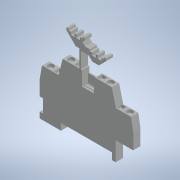
# Autodesk Inventor part: 280-519_LO
Saved by Autodesk Inventor 2021 (Build 250183000, 183)
## iProperties
Created: 2026-07-31
Part Number: 280-519_LO
Material: Generic
Catalog Web Link: www.3dfindit.com
Description: 280-519-Double-deck terminal block, Through/through terminal block, for DIN-rail 35 x 15 and 35 x 7.5, 2.5 mm², CAGE CLAMP®
Vendor: WAGO
Document SubType Name: Modeling
Designer: psAdmin
Manufacturer: WAGO
Mass: 10.061 g
Surface Area: 63.9443 cm^2
Volume: 10.5778 cm^3
Density: 1 g/cm^3
Appearance: PSOLRGB-143-145-145
Category: PARTsolutions
Company: WAGO
Title: 280-519
Author: Cadenas PARTsolutions
Comments: Double-deck terminal block, Through/through terminal block, for DIN-rail 35 x 15 and 35 x 7.5, 2.5 mm², CAGE CLAMP®
PSOL_IDENT_0: {$CADENAS_DATA/23d-libs/wago/pg01/serie280/0280-0519_0999-0962.prj},163 {VTYP=3D},{NB=280-519_LO},{L
PSOL_IDENT_1: INA=280-519},{NN=280-519},{DATE=07.07.2026 10:57:29},{GEOMDATE=12.11.2024 14:37:53},{VERSION=},{LINE
PSOL_IDENT_2: ID=2570},{WBVAR=LOD},{WBNUMERIC=}  {NB=280-519_LO},{LINA=280-519},{KT=DUMMY},{BESTNR=280-519},{INFOD
PSOL_IDENT_3: E=Info DE},{INFOEN=Info EN},{LOD=LO},{QUERSCHNITT1=0.08 - 2.5},{QUERSCHNITT2=28 - 12},{ABISOLIERLAEN
PSOL_IDENT_4: GE=8 - 9},{SPANNUNG=500},{BEMESSSTOSSSPG=6},{VERSCHMUTZGRAD=3},{STROM=20},{HOEHE=58.50},{BREITE=5.00
PSOL_IDENT_5: },{TIEFE=64.00},{ANZAHLKLEMMSTEL=4},{ANZAHLPOTENTIAL=2},{FARBE=grau},{BEMERKUNGEN=},{RGB=0.56,0.57,0
PSOL_IDENT_6: .57,0},{GEWICHT=10.061},{ECLASS71=27-14-11-20},{LINKDE=http://www.wago.com/de/p/280-519},{LINKEN=htt
PSOL_IDENT_7: p://www.wago.com/global/p/280-519},{FILENAME=280-519}
NB: 280-519_LO
NN: 280-519
NT: Double-deck terminal block, Through/through terminal block, for DIN-rail 35 x 15 and 35 x 7.5, 2.5 mm², CAGE CLAMP®
NBSYN: $BESTNR._$LOD.
LINA: 280-519
CATALOG: WAGO
OFFICIAL_STANDARD_NUMBERS: NO
BESTNR: 280-519
INFODE: Info DE
INFOEN: Info EN
LOD: LOW
QUERSCHNITT1: 0.08 - 2.5
QUERSCHNITT2: 28 - 12
ABISOLIERLAENGE: 8 - 9
SPANNUNG: 500
BEMESSSTOSSSPG: 6
VERSCHMUTZGRAD: 3
STROM: 20
HOEHE: 58.5
BREITE: 5
TIEFE: 64
ANZAHLKLEMMSTEL: 4
ANZAHLPOTENTIAL: 2
FARBE: gray
GEWICHT: 10.061
ECLASS71: 27-14-11-20
SUPPLIER: WAGO
ARTICLENO: 280-519_LO
BOMINFO: 280-519
CREATOR: CADENAS GmbH
Autodesk Inventor part; units mm, degrees
sketch "Sketch_1" plane through (0, 0, 0) normal (0, 0, 1) x (1, 0, 0)
  line L0 (-32.2, -0.6) -> (-32.2, -4.6)
  line L1 (-32.2, -4.6) -> (-17.5, -4.6)
  line L2 (-17.5, -4.6) -> (-17.5, 0)
  line L3 (-17.5, 0) -> (17.5, 0)
  line L4 (17.5, 0) -> (17.5, -4.6)
  line L5 (17.5, -4.6) -> (20, -4.6)
  line L6 (20, -4.6) -> (20, 8.5)
  line L7 (20, 8.5) -> (32, 8.5)
  line L8 (32, 8.5) -> (32, 19.1)
  line L9 (32, 19.1) -> (30.5012, 27.6)
  line L10 (30.5012, 27.6) -> (-30.5012, 27.6)
  line L11 (-30.5012, 27.6) -> (-32, 19.1)
  line L12 (-32, 19.1) -> (-32, 8.5)
  line L13 (-32, 8.5) -> (-29.7, 8.5)
  line L14 (-29.7, 8.5) -> (-29.7, -0.6)
  line L15 (-29.7, -0.6) -> (-32.2, -0.6)
  constraints: 32 end point
extrude "Extrusion1" add sketch "Sketch_1" along normal blind 5
sketch "Sketch_2" plane through (0, 0, 0) normal (0, 0, 1) x (1, 0, 0)
  line L0 (-19.1, 27.6) -> (-18.2, 27.6)
  line L1 (-18.2, 27.6) -> (-18.2, 15.1)
  line L2 (-18.2, 15.1) -> (19.2, 15.1)
  line L3 (19.2, 15.1) -> (19.2, 27.6)
  line L4 (19.2, 27.6) -> (20.1, 27.6)
  line L5 (20.1, 27.6) -> (17.3574, 38.6)
  line L6 (17.3574, 38.6) -> (5.7574, 38.6)
  line L7 (5.7574, 38.6) -> (4.9, 28.8)
  line L8 (4.9, 28.8) -> (-3.1, 28.8)
  line L9 (-3.1, 28.8) -> (-3.1, 38.6)
  line L10 (-3.1, 38.6) -> (-16.3574, 38.6)
  line L11 (-16.3574, 38.6) -> (-19.1, 27.6)
  constraints: 24 end point
extrude "Extrusion2" add sketch "Sketch_2" along normal blind 5
sketch "Skizze_3" plane through (0, 0, 0) normal (0, 0, 1) x (1, 0, 0)
  line L0 (-3.1, 34.8) -> (-3.1, 28.8)
  line L1 (-3.1, 28.8) -> (5.9, 28.8)
  line L2 (5.9, 28.8) -> (5.9, 34.8)
  line L3 (5.9, 34.8) -> (-3.1, 34.8)
  constraints: 8 end point
extrude "Extrusion3" add sketch "Skizze_3" along normal blind 0.8
sketch "Sketch_3" plane through (0.5, 0, 0) normal (1, 0, 0) x (0, 0, -1)
  line L0 (-4.7, 28.4) -> (-3.3, 28.4)
  line L1 (-3.3, 28.4) -> (-3.3, 28.8)
  line L2 (-3.3, 28.8) -> (-2.5, 28.8)
  line L3 (-2.5, 28.8) -> (-2.5, 28.4)
  line L4 (-2.5, 28.4) -> (-1.1, 28.4)
  line L5 (-1.1, 28.4) -> (-1.1, 29.8)
  line L6 (-1.1, 29.8) -> (-4.7, 29.8)
  line L7 (-4.7, 29.8) -> (-4.7, 28.4)
  constraints: 16 end point
extrude "Extrusion4" cut sketch "Sketch_3" along normal mid plane 7.2
sketch "Sketch_4" plane through (0, 0, 2.5) normal (0, 0, 1) x (1, 0, 0)
  line L0 (27.1, 25.6) -> (27.1, 27.6)
  line L1 (27.1, 27.6) -> (29.2, 27.6)
  line L2 (29.2, 27.6) -> (29.2, 25.6)
  line L3 (29.2, 25.6) -> (27.1, 25.6)
  line L4 (27.1, 25.6) -> (27.1, 27.6)
  constraints: 10 end point
revolve "Revolution1" cut sketch "Sketch_4" angle 360 about axis through (27.1, 25.6, 2.5) along (0, -1, 0)
sketch "Sketch_5" plane through (0, 0, 2.5) normal (0, 0, 1) x (1, 0, 0)
  line L0 (-27.1, 25.6) -> (-27.1, 27.6)
  line L1 (-27.1, 27.6) -> (-25, 27.6)
  line L2 (-25, 27.6) -> (-25, 25.6)
  line L3 (-25, 25.6) -> (-27.1, 25.6)
  line L4 (-27.1, 25.6) -> (-27.1, 27.6)
  constraints: 10 end point
revolve "Revolution2" cut sketch "Sketch_5" angle 360 about axis through (-27.1, 25.6, 2.5) along (0, -1, 0)
sketch "Sketch_6" plane through (0, 0, 2.5) normal (0, 0, 1) x (1, 0, 0)
  line L0 (14.05, 36.6) -> (14.05, 38.6)
  line L1 (14.05, 38.6) -> (16.15, 38.6)
  line L2 (16.15, 38.6) -> (16.15, 36.6)
  line L3 (16.15, 36.6) -> (14.05, 36.6)
  line L4 (14.05, 36.6) -> (14.05, 38.6)
  constraints: 10 end point
revolve "Revolution3" cut sketch "Sketch_6" angle 360 about axis through (14.05, 36.6, 2.5) along (0, -1, 0)
sketch "Sketch_7" plane through (0, 0, 2.5) normal (0, 0, 1) x (1, 0, 0)
  line L0 (-13.05, 36.6) -> (-13.05, 38.6)
  line L1 (-13.05, 38.6) -> (-10.95, 38.6)
  line L2 (-10.95, 38.6) -> (-10.95, 36.6)
  line L3 (-10.95, 36.6) -> (-13.05, 36.6)
  line L4 (-13.05, 36.6) -> (-13.05, 38.6)
  constraints: 10 end point
revolve "Revolution4" cut sketch "Sketch_7" angle 360 about axis through (-13.05, 36.6, 2.5) along (0, -1, 0)
sketch "Skizze_15" plane through (0, 0, 2.5) normal (0, 0, 1) x (1, 0, 0)
  line L0 (-4.9, 36.6) -> (-3.9, 36.6)
  line L1 (-3.9, 36.6) -> (-3.9, 38.6)
  line L2 (-3.9, 38.6) -> (-4.9, 38.6)
  line L3 (-4.9, 38.6) -> (-4.9, 36.6)
  constraints: 8 end point
extrude "Extrusion5" cut sketch "Skizze_15" along normal mid plane 4.1
sketch "Skizze_11" plane through (0, 0, 0.8) normal (0, 0, 1) x (1, 0, 0)
  line L0 (19.4, 25.6) -> (23, 25.6)
  line L1 (23, 25.6) -> (23, 27.6)
  line L2 (23, 27.6) -> (19.4, 27.6)
  line L3 (19.4, 27.6) -> (19.4, 25.6)
  constraints: 8 end point
extrude "Extrusion6" cut sketch "Skizze_11" along normal blind 3.6
sketch "Skizze_12" plane through (0, 0, 0.8) normal (0, 0, 1) x (1, 0, 0)
  line L0 (-23, 25.6) -> (-19.4, 25.6)
  line L1 (-19.4, 25.6) -> (-19.4, 27.6)
  line L2 (-19.4, 27.6) -> (-23, 27.6)
  line L3 (-23, 27.6) -> (-23, 25.6)
  constraints: 8 end point
extrude "Extrusion7" cut sketch "Skizze_12" along normal blind 3.6
sketch "Skizze_13" plane through (0, 0, 0.8) normal (0, 0, 1) x (1, 0, 0)
  line L0 (6.35, 36.6) -> (9.95, 36.6)
  line L1 (9.95, 36.6) -> (9.95, 38.6)
  line L2 (9.95, 38.6) -> (6.35, 38.6)
  line L3 (6.35, 38.6) -> (6.35, 36.6)
  constraints: 8 end point
extrude "Extrusion8" cut sketch "Skizze_13" along normal blind 3.6
sketch "Skizze_14" plane through (0, 0, 0.8) normal (0, 0, 1) x (1, 0, 0)
  line L0 (-8.95, 36.6) -> (-5.35, 36.6)
  line L1 (-5.35, 36.6) -> (-5.35, 38.6)
  line L2 (-5.35, 38.6) -> (-8.95, 38.6)
  line L3 (-8.95, 38.6) -> (-8.95, 36.6)
  constraints: 8 end point
extrude "Extrusion9" cut sketch "Skizze_14" along normal blind 3.6
sketch "Sketch_8" plane through (0, 0, 2.5) normal (0, 0, 1) x (1, 0, 0)
  line L0 (-13.75, 56.9029) -> (-7.4471, 50.6)
  line L1 (-7.4471, 50.6) -> (-4.9, 50.6)
  line L2 (-4.9, 50.6) -> (-4.9, 33.6)
  line L3 (-4.9, 33.6) -> (-3.9, 33.6)
  line L4 (-3.9, 33.6) -> (-3.9, 49.6)
  line L5 (-3.9, 49.6) -> (1.5103, 49.6)
  line L6 (1.5103, 49.6) -> (4.0103, 47.1)
  line L7 (4.0103, 47.1) -> (8.4471, 47.1)
  line L8 (8.4471, 47.1) -> (13.25, 51.9029)
  line L9 (13.25, 51.9029) -> (13.25, 53.6)
  line L10 (13.25, 53.6) -> (11.85, 53.6)
  line L11 (11.85, 53.6) -> (11.85, 52.45)
  line L12 (11.85, 52.45) -> (10.2, 52.45)
  line L13 (10.2, 52.45) -> (10.2, 50.6)
  line L14 (10.2, 50.6) -> (7.55, 50.6)
  line L15 (7.55, 50.6) -> (7.55, 51.3)
  line L16 (7.55, 51.3) -> (7.8, 51.3)
  line L17 (7.8, 51.3) -> (7.8, 52.8)
  line L18 (7.8, 52.8) -> (6.3, 52.8)
  line L19 (6.3, 52.8) -> (6.3, 51.3)
  line L20 (6.3, 51.3) -> (6.55, 51.3)
  line L21 (6.55, 51.3) -> (6.55, 50.6)
  line L22 (6.55, 50.6) -> (3.9, 50.6)
  line L23 (3.9, 50.6) -> (3.9, 52.45)
  line L24 (3.9, 52.45) -> (2.25, 52.45)
  line L25 (2.25, 52.45) -> (2.25, 53.6)
  line L26 (2.25, 53.6) -> (-1.0755, 53.6)
  line L27 (-1.0755, 53.6) -> (-2.8642, 55.3887)
  line L28 (-2.8642, 55.3887) -> (-1.35, 56.9029)
  line L29 (-1.35, 56.9029) -> (-1.35, 58.6)
  line L30 (-1.35, 58.6) -> (-2.75, 58.6)
  line L31 (-2.75, 58.6) -> (-2.75, 57.45)
  line L32 (-2.75, 57.45) -> (-4.4, 57.45)
  line L33 (-4.4, 57.45) -> (-4.4, 55.6)
  line L34 (-4.4, 55.6) -> (-7.05, 55.6)
  line L35 (-7.05, 55.6) -> (-7.05, 56.3)
  line L36 (-7.05, 56.3) -> (-6.8, 56.3)
  line L37 (-6.8, 56.3) -> (-6.8, 57.8)
  line L38 (-6.8, 57.8) -> (-8.3, 57.8)
  line L39 (-8.3, 57.8) -> (-8.3, 56.3)
  line L40 (-8.3, 56.3) -> (-8.05, 56.3)
  line L41 (-8.05, 56.3) -> (-8.05, 55.6)
  line L42 (-8.05, 55.6) -> (-10.7, 55.6)
  line L43 (-10.7, 55.6) -> (-10.7, 57.45)
  line L44 (-10.7, 57.45) -> (-12.35, 57.45)
  line L45 (-12.35, 57.45) -> (-12.35, 58.6)
  line L46 (-12.35, 58.6) -> (-13.75, 58.6)
  line L47 (-13.75, 58.6) -> (-13.75, 56.9029)
  constraints: 96 end point
extrude "Extrusion10" add sketch "Sketch_8" along normal mid plane 4.95
ref_plane "1_1001_XY" through (7.05, 53.6, 2.5) normal (0, 1, 0) x (-1, 0, 0)
ref_plane "1_1001_YZ" through (7.05, 53.6, 2.5) normal (-1, 0, 0) x (0, 0, 1)
ref_plane "1_1001_ZX" through (7.05, 53.6, 2.5) normal (0, 0, 1) x (0, 1, 0)
ref_plane "1_1002_XY" through (-7.55, 58.6, 2.5) normal (0, 1, 0) x (-1, 0, 0)
ref_plane "1_1002_YZ" through (-7.55, 58.6, 2.5) normal (-1, 0, 0) x (0, 0, 1)
ref_plane "1_1002_ZX" through (-7.55, 58.6, 2.5) normal (0, 0, 1) x (0, 1, 0)
ref_plane "1_13_XY" through (0.4, 28.8, 2) normal (0, 1, 0) x (-1, 0, 0)
ref_plane "1_13_YZ" through (0.4, 28.8, 2) normal (-1, 0, 0) x (0, 0, 1)
ref_plane "1_13_ZX" through (0.4, 28.8, 2) normal (0, 0, 1) x (0, 1, 0)
ref_plane "1_14_XY" through (0.4, 28.8, 3.8) normal (0, 1, 0) x (-1, 0, 0)
ref_plane "1_14_YZ" through (0.4, 28.8, 3.8) normal (-1, 0, 0) x (0, 0, 1)
ref_plane "1_14_ZX" through (0.4, 28.8, 3.8) normal (0, 0, 1) x (0, 1, 0)
ref_plane "1_2_XY" through (-21.2, 27.6, 2.6) normal (0, 1, 0) x (1, 0, 0)
ref_plane "1_2_YZ" through (-21.2, 27.6, 2.6) normal (1, 0, 0) x (0, 0, -1)
ref_plane "1_2_ZX" through (-21.2, 27.6, 2.6) normal (0, 0, -1) x (0, 1, 0)
ref_plane "1_3_XY" through (-7.15, 38.6, 2.6) normal (0, 1, 0) x (1, 0, 0)
ref_plane "1_3_YZ" through (-7.15, 38.6, 2.6) normal (1, 0, 0) x (0, 0, -1)
ref_plane "1_3_ZX" through (-7.15, 38.6, 2.6) normal (0, 0, -1) x (0, 1, 0)
ref_plane "1_4_XY" through (8.15, 38.6, 2.6) normal (0, 1, 0) x (-1, 0, 0)
ref_plane "1_4_YZ" through (8.15, 38.6, 2.6) normal (-1, 0, 0) x (0, 0, 1)
ref_plane "1_4_ZX" through (8.15, 38.6, 2.6) normal (0, 0, 1) x (0, 1, 0)
ref_plane "1_5_XY" through (21.55, 27.6, 2.6) normal (0, 1, 0) x (-1, 0, 0)
ref_plane "1_5_YZ" through (21.55, 27.6, 2.6) normal (-1, 0, 0) x (0, 0, 1)
ref_plane "1_5_ZX" through (21.55, 27.6, 2.6) normal (0, 0, 1) x (0, 1, 0)
ref_plane "1_6_XY" through (-27.1, 27.6, 2.5) normal (0, 1, 0) x (1, 0, 0)
ref_plane "1_6_YZ" through (-27.1, 27.6, 2.5) normal (1, 0, 0) x (0, 0, -1)
ref_plane "1_6_ZX" through (-27.1, 27.6, 2.5) normal (0, 0, -1) x (0, 1, 0)
ref_plane "1_7_XY" through (-13.05, 38.6, 2.5) normal (0, 1, 0) x (1, 0, 0)
ref_plane "1_7_YZ" through (-13.05, 38.6, 2.5) normal (1, 0, 0) x (0, 0, -1)
ref_plane "1_7_ZX" through (-13.05, 38.6, 2.5) normal (0, 0, -1) x (0, 1, 0)
ref_plane "1_8_XY" through (14.05, 38.6, 2.5) normal (0, 1, 0) x (-1, 0, 0)
ref_plane "1_8_YZ" through (14.05, 38.6, 2.5) normal (-1, 0, 0) x (0, 0, 1)
ref_plane "1_8_ZX" through (14.05, 38.6, 2.5) normal (0, 0, 1) x (0, 1, 0)
ref_plane "1_9_XY" through (27.1, 27.6, 2.5) normal (0, 1, 0) x (-1, 0, 0)
ref_plane "1_9_YZ" through (27.1, 27.6, 2.5) normal (-1, 0, 0) x (0, 0, 1)
ref_plane "1_9_ZX" through (27.1, 27.6, 2.5) normal (0, 0, 1) x (0, 1, 0)
ref_plane "MD_XY" through (0, 0, 0) normal (0, -1, 0) x (0, 0, 1)
ref_plane "MD_YZ" through (0, 0, 0) normal (0, 0, 1) x (-1, 0, 0)
ref_plane "MD_ZX" through (0, 0, 0) normal (-1, 0, 0) x (0, -1, 0)
ref_plane "OP_XY" through (-32.2, -4.6, 0) normal (0, 1, 0) x (0, 0, 1)
ref_plane "OP_YZ" through (-32.2, -4.6, 0) normal (0, 0, 1) x (1, 0, 0)
ref_plane "OP_ZX" through (-32.2, -4.6, 0) normal (1, 0, 0) x (0, 1, 0)
ref_plane "a1_XY" through (27.1, 12.6, 2.5) normal (0, 1, 0) x (-1, 0, 0)
ref_plane "a1_YZ" through (27.1, 12.6, 2.5) normal (-1, 0, 0) x (0, 0, 1)
ref_plane "a1_ZX" through (27.1, 12.6, 2.5) normal (0, 0, 1) x (0, 1, 0)
ref_plane "a2_XY" through (14.05, 23.6, 2.5) normal (0, 1, 0) x (-1, 0, 0)
ref_plane "a2_YZ" through (14.05, 23.6, 2.5) normal (-1, 0, 0) x (0, 0, 1)
ref_plane "a2_ZX" through (14.05, 23.6, 2.5) normal (0, 0, 1) x (0, 1, 0)
ref_plane "b3_XY" through (-13.05, 23.6, 2.5) normal (0, 1, 0) x (1, 0, 0)
ref_plane "b3_YZ" through (-13.05, 23.6, 2.5) normal (1, 0, 0) x (0, 0, -1)
ref_plane "b3_ZX" through (-13.05, 23.6, 2.5) normal (0, 0, -1) x (0, 1, 0)
ref_plane "b4_XY" through (-27.1, 12.6, 2.5) normal (0, 1, 0) x (1, 0, 0)
ref_plane "b4_YZ" through (-27.1, 12.6, 2.5) normal (1, 0, 0) x (0, 0, -1)
ref_plane "b4_ZX" through (-27.1, 12.6, 2.5) normal (0, 0, -1) x (0, 1, 0)
ref_plane "j5_XY" through (0.4, 22.8, 2) normal (0, 1, 0) x (-1, 0, 0)
ref_plane "j5_YZ" through (0.4, 22.8, 2) normal (-1, 0, 0) x (0, 0, 1)
ref_plane "j5_ZX" through (0.4, 22.8, 2) normal (0, 0, 1) x (0, 1, 0)
ref_plane "j6_XY" through (0.4, 22.8, 3.8) normal (0, 1, 0) x (-1, 0, 0)
ref_plane "j6_YZ" through (0.4, 22.8, 3.8) normal (-1, 0, 0) x (0, 0, 1)
ref_plane "j6_ZX" through (0.4, 22.8, 3.8) normal (0, 0, 1) x (0, 1, 0)
ref_plane "m7_XY" through (7.05, 53.6, 2.5) normal (0, 1, 0) x (-1, 0, 0)
ref_plane "m7_YZ" through (7.05, 53.6, 2.5) normal (-1, 0, 0) x (0, 0, 1)
ref_plane "m7_ZX" through (7.05, 53.6, 2.5) normal (0, 0, 1) x (0, 1, 0)
ref_plane "m8_XY" through (-7.55, 58.6, 2.5) normal (0, 1, 0) x (-1, 0, 0)
ref_plane "m8_YZ" through (-7.55, 58.6, 2.5) normal (-1, 0, 0) x (0, 0, 1)
ref_plane "m8_ZX" through (-7.55, 58.6, 2.5) normal (0, 0, 1) x (0, 1, 0)
ref_plane "z10_XY" through (8.15, 38.6, 2.6) normal (0, 1, 0) x (-1, 0, 0)
ref_plane "z10_YZ" through (8.15, 38.6, 2.6) normal (-1, 0, 0) x (0, 0, 1)
ref_plane "z10_ZX" through (8.15, 38.6, 2.6) normal (0, 0, 1) x (0, 1, 0)
ref_plane "z11_XY" through (-7.15, 38.6, 2.6) normal (0, 1, 0) x (1, 0, 0)
ref_plane "z11_YZ" through (-7.15, 38.6, 2.6) normal (1, 0, 0) x (0, 0, -1)
ref_plane "z11_ZX" through (-7.15, 38.6, 2.6) normal (0, 0, -1) x (0, 1, 0)
ref_plane "z12_XY" through (-21.2, 27.6, 2.6) normal (0, 1, 0) x (1, 0, 0)
ref_plane "z12_YZ" through (-21.2, 27.6, 2.6) normal (1, 0, 0) x (0, 0, -1)
ref_plane "z12_ZX" through (-21.2, 27.6, 2.6) normal (0, 0, -1) x (0, 1, 0)
ref_plane "z9_XY" through (21.55, 27.6, 2.6) normal (0, 1, 0) x (-1, 0, 0)
ref_plane "z9_YZ" through (21.55, 27.6, 2.6) normal (-1, 0, 0) x (0, 0, 1)
ref_plane "z9_ZX" through (21.55, 27.6, 2.6) normal (0, 0, 1) x (0, 1, 0)
body "Solid1"
